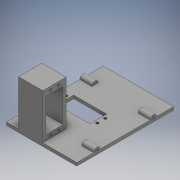
# Autodesk Inventor part: Ground_Tracker_ServoMount
Saved by Autodesk Inventor 2018 (Build 220112000, 112)
## iProperties
Created: 2018-10-21
Part Number: Ground_Tracker_ServoMount
Material: ABS Plastic
Document SubType Name: Modeling
Designer: Bradley
Density: 1.06 g/cm^3
Appearance: Smooth - Medium Gray
Author: Bradley
Autodesk Inventor part; units mm, degrees
ref_plane "YZ Plane" through (0, 0, 0) normal (1, 0, 0) x (0, 1, 0)
ref_plane "XZ Plane" through (0, 0, 0) normal (0, 1, 0) x (-1, 0, 0)
ref_plane "XY Plane" through (0, 0, 0) normal (0, 0, 1) x (1, 0, 0)
sketch "Sketch1" plane through (0, 0, 0) normal (0, 0, 1) x (1, 0, 0)
  line L0 (-30.65, -10.5) -> (10.35, -10.5)
  line L1 (10.35, -10.5) -> (10.35, 10.5)
  line L2 (10.35, 10.5) -> (-30.65, 10.5)
  line L3 (-30.65, 10.5) -> (-30.65, -10.5)
  line L4 (-30.65, -10.5) -> (10.35, 10.5) construction
  line L5 (10.35, -10.5) -> (-30.65, 10.5) construction
  line L6 (-43.65, -60) -> (43.65, -60)
  line L7 (43.65, -60) -> (43.65, 60)
  line L8 (43.65, 60) -> (-43.65, 60)
  line L9 (-43.65, 60) -> (-43.65, -60)
  line L10 (-43.65, -60) -> (43.65, 60) construction
  line L11 (43.65, -60) -> (-43.65, 60) construction
  point P0 (-10.15, 0)
  point P1 (0, 0)
  point P2 (-10.15, 0)
  point P3 (0, 0)
  dimension "d0" = 41
  dimension "d1" = 21
  dimension "d2" = 87.3
  dimension "d3" = 120
  dimension "d4" = 10.15
  constraints: 24 end point, 6 midpoint, 4 parallel, 2 horizontal, 2 perpendicular, 1 horizontal alignment
  measures "d0" distance of L2.end L1.end
  measures "d1" distance of L1.end L0.end
  measures "d2" distance of L8.end L7.end
  measures "d3" distance of L7.end L6.end
  measures "d4" distance of point (0, 0) point (-10.15, 0)
extrude "Extrusion1" add sketch "Sketch1" along normal mid plane 4
sketch "Sketch2" plane through (0, 0, 2) normal (0, 0, 1) x (1, 0, 0)
  line L0 (14, -5) -> (-34.3, -5) construction
  line L1 (-34.3, -5) -> (-34.3, 5) construction
  line L2 (-34.3, 5) -> (14, 5) construction
  line L3 (14, 5) -> (14, -5) construction
  line L4 (14, -5) -> (-34.3, 5) construction
  line L5 (-34.3, -5) -> (14, 5) construction
  point P0 (0, 0)
  point P1 (-10.15, 0)
  point P2 (-10.15, 0)
  dimension "d7" = 48.3
  dimension "d8" = 10
  dimension "d9" = 14
  constraints: 12 end point, 4 coincident, 3 midpoint, 2 parallel, 1 horizontal, 1 horizontal alignment, 1 perpendicular
  measures "d7" distance of L1.end L2.end
  measures "d8" distance of L0.end L1.end
  measures "d9" distance from line of point (0, 0) L3
hole "Hole1" at (-34.3, 5, 2) at (-34.3, -5, 2) at (14, -5, 2) at (14, 5, 2) direction (0, 0, -1) diameter 3.242 end through all thread size "M4x0.7" class "6H" standard "ANSI Metric M Profile"
sketch "Sketch3" plane through (43.65, -60, 2) normal (1, 0, 0) x (0, 0, -1)
  line L0 (4, 120) -> (0, 120) projected
  line L1 (0, 0) -> (0, 120) projected
  line L2 (4, 0) -> (0, 0) projected
  line L3 (4, 120) -> (4, 0) projected
  line L4 (0, 0) -> (0, 120) projected
  arc A0 (0, 29) -> (0, 21) centre (0, 25) ccw
  arc A1 (0, 99) -> (0, 91) centre (0, 95) ccw
  line L5 (0, 95) -> (0, 25) construction
  point P0 (2, 60)
  point P1 (0, 60)
  dimension "d17" = 70
  constraints: 6 point on line, 4 point on circle, 2 centre point, 2 end point, 2 midpoint, 2 tangent, 1 collinear
  measures "d17" distance of L5.start L5.end
extrude "Extrusion2" add sketch "Sketch3" against normal blind 15 contours L1 A1 | A0 L1
sketch "Sketch4" plane through (43.65, -60, -2) normal (1, 0, 0) x (0, 0, -1)
  line L0 (0, 120) -> (-4, 120) projected
  line L1 (-4, 99) -> (-4, 120) projected
  arc A0 (-4, 99) -> (-4, 91) centre (-4, 95) ccw projected
  line L2 (-4, 29) -> (-4, 91) projected
  arc A1 (-4, 29) -> (-4, 21) centre (-4, 25) ccw projected
  line L3 (-4, 0) -> (-4, 21) projected
  line L4 (0, 0) -> (-4, 0) projected
  line L5 (0, 120) -> (0, 0) projected
  point P0 (-2, 60)
hole "Hole2" at (43.65, 35, 2) at (43.65, -35, 2) direction (-1, 0, 0) diameter 3.242 depth 11.8 tip angle 118 thread size "M4x0.7" class "6H" standard "ANSI Metric M Profile"
mirror "Mirror1" about plane through (0, 0, 0) normal (1, 0, 0) of "Extrusion2", "Hole2"
sketch "Sketch5" plane through (0, 0, 2) normal (0, 0, 1) x (1, 0, 0)
  circle A0 centre (14, -5) radius 1.621 projected
  circle A1 centre (-34.3, 5) radius 1.621 projected
  circle A2 centre (-34.3, -5) radius 1.621 projected
  circle A3 centre (14, 5) radius 1.621 projected
  line L0 (-30.65, -10.5) -> (-30.65, 10.5) projected
  line L1 (-30.65, 10.5) -> (10.35, 10.5) projected
  line L2 (10.35, 10.5) -> (10.35, -10.5) projected
  line L3 (10.35, -10.5) -> (-30.65, -10.5) projected
  line L4 (-43.65, -31) -> (-28.65, -31) projected
  line L5 (-28.65, -31) -> (-28.65, -39) projected
  line L6 (-28.65, -39) -> (-43.65, -39) projected
  line L7 (-43.65, -39) -> (-43.65, -60) projected
  line L8 (-43.65, -60) -> (43.65, -60) projected
  line L9 (43.65, -60) -> (43.65, -39) projected
  line L10 (43.65, -39) -> (28.65, -39) projected
  line L11 (28.65, -39) -> (28.65, -31) projected
  line L12 (28.65, -31) -> (43.65, -31) projected
  line L13 (43.65, -31) -> (43.65, 31) projected
  line L14 (43.65, 31) -> (28.65, 31) projected
  line L15 (28.65, 31) -> (28.65, 39) projected
  line L16 (28.65, 39) -> (43.65, 39) projected
  line L17 (43.65, 39) -> (43.65, 60) projected
  line L18 (43.65, 60) -> (-43.65, 60) projected
  line L19 (-43.65, 60) -> (-43.65, 39) projected
  line L20 (-43.65, 39) -> (-28.65, 39) projected
  line L21 (-28.65, 39) -> (-28.65, 31) projected
  line L22 (-28.65, 31) -> (-43.65, 31) projected
  line L23 (-43.65, 31) -> (-43.65, -31) projected
  line L24 (-28.65, -35) -> (1.35, -35)
  line L25 (1.35, -35) -> (1.35, -56)
  line L26 (1.35, -56) -> (-28.65, -56)
  line L27 (-28.65, -56) -> (-28.65, -35)
  line L28 (-28.65, -31) -> (-28.65, -39) projected
  line L29 (10.35, 10.5) -> (10.35, -10.5) projected
  point P0 (0, 0)
  dimension "d27" = 45
  dimension "d28" = 4
  constraints: 8 end point, 3 parallel, 1 collinear, 1 horizontal, 1 perpendicular
  measures "d27" distance between parallel lines of L23 L25
  measures "d28" distance between parallel lines of L8 L26
extrude "Extrusion3" add sketch "Sketch5" along normal blind 7 contours L24 L25 L26 L27 L5
sketch "Sketch6" plane through (1.35, -56, 2) normal (1, 0, 0) x (0, 0, -1)
  line L0 (0, 21) -> (0, 0) projected
  line L1 (0, 21) -> (-7, 21) projected
  line L2 (-7, 0) -> (-7, 21) projected
  line L3 (0, 0) -> (-7, 0) projected
  line L4 (-56, -4) -> (0, -4)
  line L5 (0, -4) -> (0, 25)
  line L6 (0, 25) -> (-56, 25)
  line L7 (-56, 25) -> (-56, -4)
  line L8 (-7, 0) -> (-48, 0)
  line L9 (-48, 0) -> (-48, 21)
  line L10 (-48, 21) -> (-7, 21)
  line L11 (-7, 21) -> (-7, 0)
  line L12 (0, 25) -> (0, 87) projected
  line L13 (0, -4) -> (4, -4) projected
  point P0 (2, 56)
  point P1 (0, 10.5)
  dimension "d31" = 41
  dimension "d32" = 8
  constraints: 16 end point, 4 parallel, 2 collinear, 2 horizontal, 2 midpoint, 2 perpendicular
  measures "d31" distance of L2.start L8.end
  measures "d32" distance between parallel lines of L9 L7
extrude "Extrusion4" add sketch "Sketch6" against normal up to surface (30 mm away) contours L0 L3 L2 L1 | L1 L10 L9 L8 L3 L5 L4 L7 L6
sketch "Sketch8" plane through (1.35, -60, 58) normal (1, 0, 0) x (0, 0, -1)
  line L0 (56, 29) -> (56, 0) projected
  line L1 (4.35, 9.5) -> (52.65, 9.5) construction
  line L2 (52.65, 9.5) -> (52.65, 19.5) construction
  line L3 (52.65, 19.5) -> (4.35, 19.5) construction
  line L4 (4.35, 19.5) -> (4.35, 9.5) construction
  line L5 (56, 29) -> (0, 29) projected
  line L6 (0, 29) -> (0, 0) projected
  line L7 (0, 0) -> (56, 0) projected
  point P0 (58, 60)
  point P1 (4.35, 14.5)
  point P2 (8, 14.5)
  point P3 (28.5, 19.5)
  point P4 (28.5, 25)
  dimension "d38" = 48.3
  dimension "d39" = 10
  constraints: 8 end point, 4 coincident, 2 midpoint, 2 parallel, 1 horizontal, 1 horizontal alignment, 1 perpendicular, 1 vertical alignment
  measures "d38" distance of L1.start L1.end
  measures "d39" distance of L3.end L1.start
hole "Hole3" at (1.35, -50.5, 53.65) at (1.35, -40.5, 53.65) at (1.35, -40.5, 5.35) at (1.35, -50.5, 5.35) direction (-1, 0, 0) diameter 3.242 depth 11.8 tip angle 118 thread size "M4x0.7" class "6H" standard "ANSI Metric M Profile"
body "Solid1"
